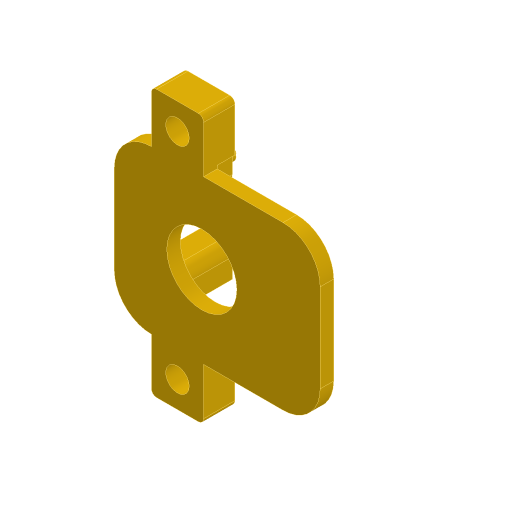
# Autodesk Inventor part: PrzyciskSTOP_2
Saved by Autodesk Inventor 2024.3 (Build 283343000, 343)
## iProperties
Created: 2025-08-19
Part Number: PrzyciskSTOP_2
Material: Generic
Document SubType Name: Modeling
Designer: PM
Density: 1 g/cm^3
Appearance: Gold
Author: PM
## iProperties of the stored document PrzyciskSTOP_2_3DPrint.ipt
Created: 2025-08-19
Part Number: PrzyciskSTOP_2_3DPrint
Material: Generic
Document SubType Name: Modeling
Designer: PM
Density: 1 g/cm^3
Appearance: Default
Author: PM
Autodesk Inventor part; units mm, degrees
ref_plane "YZ Plane" through (0, 0, 0) normal (1, 0, 0) x (0, 1, 0)
ref_plane "Work Plane1" through (0, 0, 0.6) normal (0, 0, 1) x (1, 0, 0)
sketch "Sketch1" plane through (0, 0, 0.6) normal (0, 0, 1) x (1, 0, 0)
  circle A0 centre (-11.825, -7.675) radius 1.2 projected
  circle A1 centre (-11.825, 7.675) radius 1.2 projected
  line L0 (-14.7, 10.55) -> (-8.95, 10.55)
  line L1 (-8.95, 10.55) -> (-8.95, 4.8)
  line L2 (-8.95, 4.8) -> (-14.7, 4.8)
  line L3 (-14.7, 4.8) -> (-14.7, 10.55)
  line L4 (-14.7, 10.55) -> (-8.95, 4.8) construction
  line L5 (-8.95, 10.55) -> (-14.7, 4.8) construction
  line L6 (-14.7, -10.55) -> (-8.95, -10.55)
  line L7 (-8.95, -10.55) -> (-8.95, -4.8)
  line L8 (-8.95, -4.8) -> (-14.7, -4.8)
  line L9 (-14.7, -4.8) -> (-14.7, -10.55)
  line L10 (-14.7, -10.55) -> (-8.95, -4.8) construction
  line L11 (-8.95, -10.55) -> (-14.7, -4.8) construction
  arc A2 (-19.7, -8.45) -> (-12.6, -15.55) centre (-12.6, -8.45) ccw projected
  line L12 (-12.6, -15.55) -> (12.6, -15.55) projected
  arc A3 (12.6, -15.55) -> (19.7, -8.45) centre (12.6, -8.45) ccw projected
  line L13 (19.7, -8.45) -> (19.7, -7) projected
  line L14 (19.7, -7) -> (15.7, -7) projected
  line L15 (15.7, -7) -> (15.7, -8.45) projected
  arc A4 (12.6, -11.55) -> (15.7, -8.45) centre (12.6, -8.45) ccw projected
  line L16 (12.6, -11.55) -> (-12.6, -11.55) projected
  arc A5 (-15.7, -8.45) -> (-12.6, -11.55) centre (-12.6, -8.45) ccw projected
  line L17 (-15.7, -8.45) -> (-15.7, 8.45) projected
  arc A6 (-12.6, 11.55) -> (-15.7, 8.45) centre (-12.6, 8.45) ccw projected
  line L18 (-12.6, 11.55) -> (12.6, 11.55) projected
  arc A7 (15.7, 8.45) -> (12.6, 11.55) centre (12.6, 8.45) ccw projected
  line L19 (15.7, 8.45) -> (15.7, 7) projected
  line L20 (15.7, 7) -> (19.7, 7) projected
  line L21 (19.7, 7) -> (19.7, 8.45) projected
  arc A8 (19.7, 8.45) -> (12.6, 15.55) centre (12.6, 8.45) ccw projected
  line L22 (12.6, 15.55) -> (-12.6, 15.55) projected
  arc A9 (-12.6, 15.55) -> (-19.7, 8.45) centre (-12.6, 8.45) ccw projected
  line L23 (-19.7, 8.45) -> (-19.7, -8.45) projected
  point P0 (0, 0)
  dimension "d1" = 1
  dimension "d2" = 1
  constraints: 24 end point, 4 midpoint, 4 parallel, 2 equal length, 2 horizontal, 2 perpendicular
  measures "d1" distance between parallel lines of L18 L0
  measures "d2" distance between parallel lines of L17 L3
ref_plane "Work Plane2" through (-15.1, -10.95, -8.65) normal (0, 0, 1) x (1, 0, 0)
extrude "Extrusion1" add sketch "Sketch1" against normal up to surface (9.25 mm away) contours A0 | A1 | L0 L1 L2 L3 | L9 L8 L7 L6
fillet "Fillet1" radius 2 4 edges at (-14.7, 10.55, -4.025) (-14.7, -10.55, -4.025) (-8.95, 4.8, -4.025) (-8.95, -4.8, -4.025)
sketch "Sketch2" plane through (-10.95, 4.8, -8.65) normal (0, 0, -1) x (-1, 0, 0)
  circle A0 centre (0.875, 2.875) radius 1.2 projected
  circle A1 centre (0.875, -12.475) radius 1.2 projected
  point P0 (-10.95, -4.8)
extrude "Extrusion2" add sketch "Sketch2" along normal blind 3
chamfer "Chamfer1" distance 0.6 angle 45 2 edges at (-10.625, 7.675, -11.65) (-10.625, -7.675, -11.65)
sketch "Sketch3" plane through (0, 0, 0.6) normal (0, 0, 1) x (1, 0, 0)
  arc A0 (-19.7, -8.45) -> (-12.6, -15.55) centre (-12.6, -8.45) ccw projected
  line L0 (-12.6, -15.55) -> (12.6, -15.55) projected
  arc A1 (12.6, -15.55) -> (19.7, -8.45) centre (12.6, -8.45) ccw projected
  line L1 (19.7, -8.45) -> (19.7, -7) projected
  line L2 (19.7, -7) -> (15.7, -7) projected
  line L3 (15.7, -7) -> (15.7, -8.45) projected
  arc A2 (12.6, -11.55) -> (15.7, -8.45) centre (12.6, -8.45) ccw projected
  line L4 (12.6, -11.55) -> (-12.6, -11.55) projected
  arc A3 (-15.7, -8.45) -> (-12.6, -11.55) centre (-12.6, -8.45) ccw projected
  line L5 (-15.7, -8.45) -> (-15.7, 8.45) projected
  arc A4 (-12.6, 11.55) -> (-15.7, 8.45) centre (-12.6, 8.45) ccw projected
  line L6 (-12.6, 11.55) -> (12.6, 11.55) projected
  arc A5 (15.7, 8.45) -> (12.6, 11.55) centre (12.6, 8.45) ccw projected
  line L7 (15.7, 8.45) -> (15.7, 7) projected
  line L8 (15.7, 7) -> (19.7, 7) projected
  line L9 (19.7, 7) -> (19.7, 8.45) projected
  arc A6 (19.7, 8.45) -> (12.6, 15.55) centre (12.6, 8.45) ccw projected
  line L10 (12.6, 15.55) -> (-12.6, 15.55) projected
  arc A7 (-12.6, 15.55) -> (-19.7, 8.45) centre (-12.6, 8.45) ccw projected
  line L11 (-19.7, 8.45) -> (-19.7, -8.45) projected
  circle A8 centre (-11.825, 7.675) radius 1.2 projected
  circle A9 centre (-11.825, -7.675) radius 1.2 projected
  line L12 (19.7, 7) -> (15.7, 7) projected
  line L13 (15.7, 7) -> (15.7, 8.45) projected
  arc A10 (15.7, 8.45) -> (12.6, 11.55) centre (12.6, 8.45) ccw projected
  line L14 (12.6, 11.55) -> (-12.6, 11.55) projected
  arc A11 (-12.6, 11.55) -> (-15.7, 8.45) centre (-12.6, 8.45) ccw projected
  line L15 (-15.7, 8.45) -> (-15.7, -8.45) projected
  arc A12 (-15.7, -8.45) -> (-12.6, -11.55) centre (-12.6, -8.45) ccw projected
  line L16 (-12.6, -11.55) -> (12.6, -11.55) projected
  arc A13 (12.6, -11.55) -> (15.7, -8.45) centre (12.6, -8.45) ccw projected
  line L17 (15.7, -8.45) -> (15.7, -7) projected
  line L18 (15.7, -7) -> (19.7, -7) projected
  line L19 (19.7, 7) -> (19.7, -7) projected
  line L20 (15.7, -7) -> (15.7, 7)
  point P0 (0, 0)
  constraints: 2 end point, 1 collinear
extrude "Extrusion3" add sketch "Sketch3" along normal blind 2.6 contours L11 A7 L10 A6 L9 L8 L7 A5 L6 A4 L5 A3 L4 A2 L3 L2 L1 A1 L0 A0 | L2 L20 L8 L19 | L3 A2 L4 A3 L5 A4 L6 A5 L7 L20 | A8 | A9
sketch "Sketch4" plane through (0, 0, 3.2) normal (0, 0, 1) x (1, 0, 0)
  circle A0 centre (-2.95, 0) radius 5.7 projected
  circle A1 centre (-2.95, 0) radius 6.7
  point P0 (0, 0)
  dimension "d13" = 1
  constraints: 1 centre point
  measures "d13" radial gap between concentric circles of A0 A1
extrude "Extrusion4" cut sketch "Sketch4" against normal through all contours A0 | A1
sketch "Sketch5" plane through (0, 0, 3.2) normal (0, 0, 1) x (1, 0, 0)
  circle A0 centre (-2.95, 0) radius 6.7 projected
  line L0 (19.7, -8.45) -> (19.7, 8.45) projected
  arc A1 (19.7, 8.45) -> (12.6, 15.55) centre (12.6, 8.45) ccw projected
  line L1 (12.6, 15.55) -> (-12.6, 15.55) projected
  arc A2 (-12.6, 15.55) -> (-19.7, 8.45) centre (-12.6, 8.45) ccw projected
  line L2 (-19.7, 8.45) -> (-19.7, -8.45) projected
  arc A3 (-19.7, -8.45) -> (-12.6, -15.55) centre (-12.6, -8.45) ccw projected
  line L3 (-12.6, -15.55) -> (12.6, -15.55) projected
  arc A4 (12.6, -15.55) -> (19.7, -8.45) centre (12.6, -8.45) ccw projected
  arc A5 (-12.6, -24.55) -> (-11.6, -25.55) centre (-11.6, -24.55) ccw projected
  line L4 (-11.6, -25.55) -> (-3.6, -25.55) projected
  arc A6 (-3.6, -25.55) -> (-2.6, -24.55) centre (-3.6, -24.55) ccw projected
  line L5 (-2.6, -24.55) -> (-2.6, -16.55) projected
  arc A7 (-1.6, -15.55) -> (-2.6, -16.55) centre (-1.6, -16.55) ccw projected
  line L6 (-1.6, -15.55) -> (-12.6, -15.55) projected
  arc A8 (-13.4765, -15.4957) -> (-12.6, -15.55) centre (-12.6, -8.45) ccw projected
  arc A9 (-12.6, -16.488) -> (-13.4765, -15.4957) centre (-13.6, -16.488) ccw projected
  line L7 (-12.6, -16.488) -> (-12.6, -24.55) projected
  circle A10 centre (-7.6, -20.55) radius 2.25 projected
  arc A11 (-2.6, 24.55) -> (-3.6, 25.55) centre (-3.6, 24.55) ccw projected
  line L8 (-3.6, 25.55) -> (-11.6, 25.55) projected
  arc A12 (-11.6, 25.55) -> (-12.6, 24.55) centre (-11.6, 24.55) ccw projected
  line L9 (-12.6, 24.55) -> (-12.6, 16.488) projected
  arc A13 (-13.4765, 15.4957) -> (-12.6, 16.488) centre (-13.6, 16.488) ccw projected
  arc A14 (-12.6, 15.55) -> (-13.4765, 15.4957) centre (-12.6, 8.45) ccw projected
  line L10 (-1.6, 15.55) -> (-12.6, 15.55) projected
  arc A15 (-2.6, 16.55) -> (-1.6, 15.55) centre (-1.6, 16.55) ccw projected
  line L11 (-2.6, 16.55) -> (-2.6, 24.55) projected
  circle A16 centre (-7.6, 20.55) radius 2.25 projected
  line L12 (-12.6, -16.488) -> (-12.6, -15.55)
  line L13 (-2.6, -16.55) -> (-2.6, -15.55)
  line L14 (-12.6, 16.488) -> (-12.6, 15.55)
  line L15 (-2.6, 16.55) -> (-2.6, 15.55)
  point P0 (0, 0)
  constraints: 8 end point, 2 perpendicular, 2 point on line, 2 vertical, 1 tangent
extrude "Extrusion5" add sketch "Sketch5" against normal blind 6 contours L13 L5 A6 L4 A5 L7 L12 L3 | L1 L14 L9 A12 L8 A11 L11 L15
sketch "Sketch6" plane through (-12.6, 15.55, 0.6) normal (0, -1, 0) x (1, 0, 0)
  line L0 (10, 0) -> (0, 0) projected
  line L1 (0, 0) -> (0, -3.4) projected
  line L2 (10, -3.4) -> (0, -3.4) projected
  line L3 (10, 0) -> (10, -3.4) projected
  point P0 (12.6, -0.6)
extrude "Extrusion6" cut sketch "Sketch6" against normal blind 0.6
mirror "Mirror1" about plane through (0, 0, 0) normal (0, 1, 0) of "Extrusion6"
equation "\"d2\" = d1"
body "Solid1"
